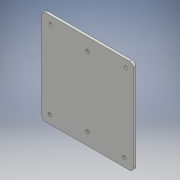
# Autodesk Inventor part: nuc_case_top
Saved by Autodesk Inventor 2018 (Build 220112000, 112)
## iProperties
Created: 2017-11-18
Part Number: nuc_case_top
Material: Genérico
Document SubType Name: Modeling
Designer: se_ma
Density: 1 g/cm^3
Appearance: Valor por defecto
Author: se_ma
Autodesk Inventor part; units mm, degrees
ref_plane "YZ Plane" through (0, 0, 0) normal (1, 0, 0) x (0, 1, 0)
ref_plane "XZ Plane" through (0, 0, 0) normal (0, 1, 0) x (-1, 0, 0)
ref_plane "XY Plane" through (0, 0, 0) normal (0, 0, 1) x (1, 0, 0)
sketch "Boceto1" plane through (0, 0, 0) normal (0, 1, 0) x (-1, 0, 0)
  line L0 (0, -5) -> (0, -110)
  line L1 (-5, -115) -> (-107, -115)
  line L2 (-112, -110) -> (-112, -5)
  line L3 (-107, 0) -> (-5, 0)
  arc A0 (-5, -115) -> (0, -110) centre (-5, -110) ccw
  arc A1 (-107, 0) -> (-112, -5) centre (-107, -5) ccw
  arc A2 (-112, -110) -> (-107, -115) centre (-107, -110) ccw
  arc A3 (0, -5) -> (-5, 0) centre (-5, -5) ccw
  circle A4 centre (-10, -105) radius 2
  circle A5 centre (-101, -105) radius 2
  circle A6 centre (-103, -9) radius 2
  circle A7 centre (-11, -9) radius 2
  point P0 (0, 0)
  dimension "d2" = 5
  dimension "d3" = 5
  dimension "d21" = 4
  dimension "d24" = 4
  dimension "d27" = 4
  dimension "d30" = 4
  constraints: 8 centre point, 8 end point, 8 point on circle, 8 tangent, 2 equal radius, 2 parallel, 1 perpendicular
  measures "d2" radius of A0
  measures "d3" radius of A2
  measures "d21" diameter of A4
  measures "d24" diameter of A5
  measures "d27" diameter of A6
  measures "d30" diameter of A7
extrude "Extrusión1" add sketch "Boceto1" along normal blind 3
sketch "Boceto2" plane through (0, 3, 0) normal (0, 1, 0) x (1, 0, 0)
  line L0 (5, 0) -> (107, 0) projected
  line L1 (107, 115) -> (5, 115) projected
  line L2 (58.3094, 19) -> (60.6188, 15)
  line L3 (60.6188, 15) -> (58.3094, 11)
  line L4 (58.3094, 11) -> (53.6906, 11)
  line L5 (53.6906, 11) -> (51.3812, 15)
  line L6 (51.3812, 15) -> (53.6906, 19)
  line L7 (53.6906, 19) -> (58.3094, 19)
  line L8 (53.6906, 96) -> (51.3812, 100)
  line L9 (51.3812, 100) -> (53.6906, 104)
  line L10 (53.6906, 104) -> (58.3094, 104)
  line L11 (58.3094, 104) -> (60.6188, 100)
  line L12 (60.6188, 100) -> (58.3094, 96)
  line L13 (58.3094, 96) -> (53.6906, 96)
  line L14 (66, 57.5) -> (66, 12.5)
  line L15 (61, 7.5) -> (51, 7.5)
  line L16 (46, 12.5) -> (46, 102.5)
  line L17 (51, 107.5) -> (61, 107.5)
  line L18 (66, 102.5) -> (66, 57.5)
  arc A0 (46, 12.5) -> (51, 7.5) centre (51, 12.5) ccw
  arc A1 (61, 7.5) -> (66, 12.5) centre (61, 12.5) ccw
  arc A2 (66, 102.5) -> (61, 107.5) centre (61, 102.5) ccw
  arc A3 (51, 107.5) -> (46, 102.5) centre (51, 102.5) ccw
  point P0 (0, 0)
  point P1 (56, 15)
  point P2 (56, 100)
  point P3 (66, 107.5)
  dimension "d42" = 5
  constraints: 34 end point, 8 point on circle, 8 tangent, 4 centre point, 4 perpendicular, 3 equal radius, 3 point on line, 1 vertical, 26 other
  measures "d42" radius of A0
extrude "Extrusión2" add sketch "Boceto2" along normal blind 3
sketch "Boceto3" plane through (0, 3, 0) normal (0, 1, 0) x (1, 0, 0)
  line L0 (53.6906, 19) -> (58.3094, 19) projected
  line L1 (58.3094, 104) -> (53.6906, 104) projected
  circle A0 centre (56, 15) radius 2
  circle A1 centre (56, 100) radius 2
  point P0 (0, 0)
  dimension "d45" = 4
  dimension "d46" = 4
  constraints: 2 centre point
  measures "d45" diameter of A0
  measures "d46" diameter of A1
extrude "Extrusión3" cut sketch "Boceto3" against normal blind 3
